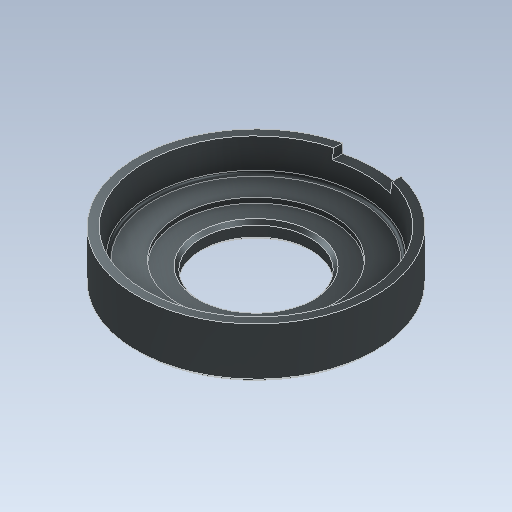
# Autodesk Inventor part: Корпус маслосъемника_CPY
Saved by Autodesk Inventor 2021 (Build 250183000, 183)
## iProperties
Created: 2020-11-17
Part Number: Корпус маслосъемника_CPY
Material: Чугун, серый
Document SubType Name: Modeling
Designer: Тимоха
Mass: 1884.24 g
Surface Area: 577.366 cm^2
Volume: 263.531 cm^3
Density: 7.15 g/cm^3
Appearance: Чугун серый
Author: Тимоха
Autodesk Inventor part; units mm, degrees
ref_plane "YZ Plane" through (0, 0, 0) normal (1, 0, 0) x (0, 1, 0)
ref_plane "XZ Plane" through (0, 0, 0) normal (0, 1, 0) x (-1, 0, 0)
ref_plane "XY Plane" through (0, 0, 0) normal (0, 0, 1) x (1, 0, 0)
sketch "Эскиз1" plane through (0, 0, 0) normal (0, 0, 1) x (1, 0, 0)
  line L0 (0, 0) -> (70, 0)
  line L1 (70, 0) -> (70, 30)
  line L2 (70, 30) -> (65, 30)
  line L3 (32, 13) -> (32, 0)
  line L4 (65, 30) -> (61.7485, 13)
  line L5 (0, -6) -> (0, 36) projected
  line L6 (32, 13) -> (61.7485, 13)
  dimension "d0" = 70
  dimension "d1" = 30
  dimension "d2" = 5
  dimension "d16" = 32
  constraints: 12 end point, 3 perpendicular, 2 horizontal, 1 point on line
  measures "d0" distance of L0.start L0.end
  measures "d1" distance of L0.end L1.end
  measures "d2" distance of L1.end L2.end
  measures "d16" distance between parallel lines of L3 L5
revolve "Вращение1" add sketch "Эскиз1" angle 360 about axis through (0, -10, 0) along (0, 1, 0)
sketch "Эскиз2" plane through (0, 13, 0) normal (0, 1, 0) x (1, 0, 0)
  circle A0 centre (0, 0) radius 45
  circle A1 centre (0, 0) radius 32 projected
  dimension "d6" = 90
  constraints: 1 centre point, 1 coincident
  measures "d6" diameter of A0
extrude "Выдавливание1" cut sketch "Эскиз2" against normal blind 3
chamfer "Фаска1" distance 2 angle 45 2 edges at (-32, 10, 0) (-32, 0, 0)
chamfer "Фаска2" distance 2 angle 45 1 edges at (-70, 0, 0)
fillet "Сопряжение1" radius 2 1 edges at (-61.7485, 13, 0)
sketch "Эскиз3" plane through (0, 0, 0) normal (0, 0, 1) x (1, 0, 0)
  line L0 (0, 0) -> (0, -10)
  line L1 (-17.039, 24.5) -> (-17.039, 30)
  line L2 (17.039, 24.5) -> (-17.039, 24.5)
  line L3 (0, -18.3) -> (0, 39.8) projected
  line L4 (0, 30) -> (17.039, 30)
  line L5 (-70, 30) -> (70, 30) projected
  line L6 (17.039, 30) -> (17.039, 24.5)
  line L7 (0, 30) -> (-17.039, 30)
  constraints: 12 end point, 3 point on line, 1 symmetric about line, 1 vertical
extrude "Выдавливание2" cut sketch "Эскиз3" against normal through all
